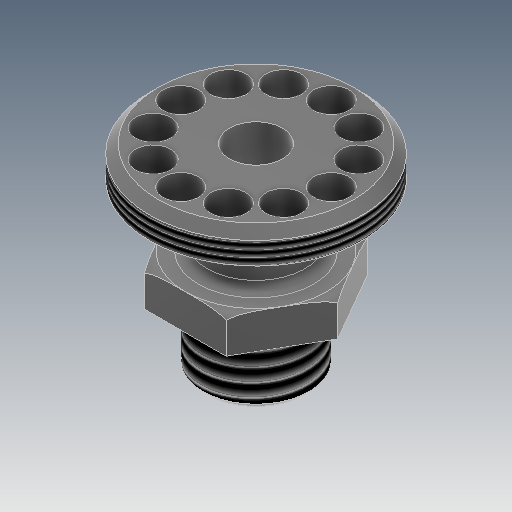
# Autodesk Inventor part: 通气器主体
Saved by Autodesk Inventor 2025 (Build 290162000, 162)
## iProperties
Created: 2025-03-16
Part Number: 通气器主体
Material: 钢，软
Document SubType Name: Modeling
Designer: ASUS
Density: 7.85 g/cm^3
Appearance: 平滑 - 黑色
Author: ASUS
Autodesk Inventor part; units mm, degrees
ref_plane "YZ Plane" through (0, 0, 0) normal (1, 0, 0) x (0, 1, 0)
ref_plane "XZ Plane" through (0, 0, 0) normal (0, 1, 0) x (-1, 0, 0)
ref_plane "XY Plane" through (0, 0, 0) normal (0, 0, 1) x (1, 0, 0)
sketch "草图2" plane through (0, 0, 0) normal (1, 0, 0) x (0, 1, 0)
  line L0 (0, 0) -> (0, 22)
  line L1 (0, 22) -> (-2, 24)
  line L2 (-2, 24) -> (-7, 24)
  line L3 (-7, 24) -> (-7, 11)
  line L4 (-7, 11) -> (-21, 11)
  line L5 (-21, 11) -> (-21, 18.45)
  line L6 (-21, 18.45) -> (-29, 18.45)
  line L7 (-29, 18.45) -> (-29, 11)
  line L8 (-29, 11) -> (-30.5, 11)
  line L9 (-30.5, 11) -> (-30.5, 12)
  line L10 (-30.5, 12) -> (-42.5, 12)
  line L11 (-42.5, 12) -> (-44, 10.5)
  line L12 (-44, 10.5) -> (-44, 0)
  line L13 (-44, 0) -> (0, 0)
  line L14 (0, 6) -> (-44, 6)
  arc A0 (-21, 15.952238) -> (-22, 18.45) centre (-24.619408, 15.952238) ccw
  dimension "d0" = 6
  dimension "d5" = 12
  dimension "d6" = 1
  dimension "d7" = 18.45
  dimension "d8" = 11
  dimension "d9" = 24
  dimension "d10" = 45
  dimension "d11" = 1.5
  dimension "d12" = 2
  dimension "d13" = 7
  dimension "d14" = 8
  dimension "d15" = 22
  dimension "d16" = 15
  dimension "d17" = 1.5
  constraints: 30 end point, 12 perpendicular, 4 point on line, 2 point on circle, 1 centre point, 1 parallel, 1 tangent, 1 vertical
  measures "d0" distance between parallel lines of L13 L14
  measures "d5" distance between parallel lines of L13 L10
  measures "d6" distance of L8.end L9.end
  measures "d7" distance between parallel lines of L13 L6
  measures "d8" distance between parallel lines of L13 L4
  measures "d9" distance between parallel lines of L13 L2
  measures "d10" angle of L10 L11
  measures "d11" distance from line of L11.end L10
  measures "d12" distance from line of L2 L0.end
  measures "d13" distance between parallel lines of L3 L0
  measures "d14" distance between parallel lines of L7 L5
  measures "d15" distance between parallel lines of L3 L7
  measures "d16" distance between parallel lines of L12 L7
  measures "d17" distance of L7.end L8.end
revolve "旋转1" add sketch "草图2" angle 360 about axis through (0, -44, 0) along (0, 1, 0) contours L14 L12 L11 L10 L9 L8 L7 L6 A0 L5 L4 L3 L2 L1 L0
fillet "圆角1" radius 2 2 edges at (0, -21, -11) (0, -7, -11)
sketch "草图3" plane through (0, -29, 0) normal (0, -1, 0) x (1, 0, 0)
  circle A0 centre (0, 0) radius 18.45
  line L0 (18.45, 0) -> (9.225, -15.978169)
  line L1 (9.225, -15.978169) -> (-9.225, -15.978169)
  line L2 (-9.225, -15.978169) -> (-18.45, 0)
  line L3 (-18.45, 0) -> (-9.225, 15.978169)
  line L4 (-9.225, 15.978169) -> (9.225, 15.978169)
  line L5 (9.225, 15.978169) -> (18.45, 0)
  point P0 (-18.45, 0)
  point P1 (-18.45, 0)
  constraints: 12 end point, 1 coincident, 15 other
extrude "拉伸1" cut sketch "草图3" against normal up to surface (8 mm away) contours L5 A0 | A0 L0 | L4 A0 | A0 L1 | L3 A0 | A0 L2
thread "螺纹1" size "M24x3" designation "M24" class "6g" standard "GB Metric profile" length 20
thread "螺纹2" size "M48x1.5" class "6g" standard "GB Metric profile" length 20
sketch "草图4" plane through (0, 0, 0) normal (0, 1, 0) x (1, 0, 0)
  circle A0 centre (0, 0) radius 13
  circle A1 centre (0, -17) radius 4
  circle A2 centre (8.5, -14.722432) radius 4
  circle A3 centre (14.722432, -8.5) radius 4
  circle A4 centre (17, 0) radius 4
  circle A5 centre (14.722432, 8.5) radius 4
  circle A6 centre (8.5, 14.722432) radius 4
  circle A7 centre (0, 17) radius 4
  circle A8 centre (-8.5, 14.722432) radius 4
  circle A9 centre (-14.722432, 8.5) radius 4
  circle A10 centre (-17, 0) radius 4
  circle A11 centre (-14.722432, -8.5) radius 4
  circle A12 centre (-8.5, -14.722432) radius 4
  point P0 (0, 0)
  dimension "d26" = 8
  dimension "d27" = 17
  dimension "d30" = 360
  constraints: 12 centre point, 25 other
  measures "d26" diameter of A1
  measures "d27" distance of A1.centre point (0, 0)
extrude "拉伸2" cut sketch "草图4" against normal up to next contours A3 | A2 | A1 | A12 | A11 | A10 | A9 | A8 | A7 | A6 | A5 | A4
equation "\"d0\" = 0.5 * d2"
equation "\"d5\" = 0.5 * d"
equation "\"d7\" = 0.5 * D1"
equation "\"d8\" = 0.5 * d4"
equation "\"d9\" = 0.5 * d1"
equation "\"d13\" = K_"
equation "\"d14\" = b"
equation "\"d15\" = h1"
equation "\"d16\" = a"
equation "\"d\" = 24"
equation "\"d1\" = 48"
equation "\"d2\" = 12"
equation "\"d3\" = 5"
equation "\"d4\" = 22"
equation "\"D\" = 55"
equation "\"a\" = 15"
equation "\"b\" = 8"
equation "\"h1\" = 22"
equation "\"D1\" = 36.9"
equation "\"S_\" = 32"
equation "\"K_\" = 7"
equation "\"e\" = 2"
equation "\"f_\" = 2"
